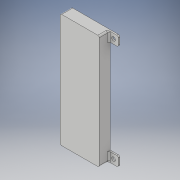
# Autodesk Inventor part: Supporter
Saved by Autodesk Inventor 2018 (Build 220112000, 112)
## iProperties
Created: 2017-12-13
Part Number: Supporter
Material: Generic
Document SubType Name: Modeling
Designer: kcmat
Density: 1 g/cm^3
Appearance: Default
Author: kcmat
Autodesk Inventor part; units mm, degrees
ref_plane "YZ Plane" through (0, 0, 0) normal (1, 0, 0) x (0, 1, 0)
ref_plane "XZ Plane" through (0, 0, 0) normal (0, 1, 0) x (-1, 0, 0)
sketch "Sketch1" plane through (0, 0, 0) normal (0, 0, 1) x (1, 0, 0)
  line L0 (165.7182, 252.0837) -> (146.6642, 252.0837) projected
  line L1 (158.6327, 216.5237) -> (165.7182, 216.5237) projected
  line L2 (139.5562, 216.5237) -> (143.6242, 216.5237) projected
  line L3 (143.6242, 252.0837) -> (139.5562, 252.0837) projected
  line L4 (126.4117, 267.0247) -> (136.1907, 267.0247) projected
  line L5 (136.1907, 190.8247) -> (126.4117, 190.8247) projected
  line L6 (139.5562, 267.0247) -> (139.5562, 190.8247)
  line L7 (139.5562, 190.8247) -> (165.7182, 190.8247)
  line L8 (165.7182, 190.8247) -> (165.7182, 267.0247)
  line L9 (165.7182, 267.0247) -> (139.5562, 267.0247)
  point P0 (0, 0)
  constraints: 8 end point, 3 perpendicular, 1 vertical
ref_plane "Work Plane1" through (146.6642, 216.5237, 7.3936) normal (0, 0, -1) x (0, 1, 0)
extrude "Extrusion1" add sketch "Sketch1" along normal up to surface (7.3936 mm away)
sketch "Sketch2" plane through (0, 0, 0) normal (0, 0, -1) x (-1, 0, 0)
  line L0 (-165.7182, 267.0247) -> (-139.5562, 267.0247) projected
  line L1 (-165.7182, 267.0247) -> (-172.0682, 267.0247)
  line L2 (-172.0682, 267.0247) -> (-172.0682, 260.6747)
  line L3 (-172.0682, 260.6747) -> (-165.7182, 260.6747)
  line L4 (-165.7182, 190.8247) -> (-165.7182, 267.0247) projected
  circle A0 centre (-168.8932, 263.8497) radius 1.25
  line L5 (-165.7182, 228.9247) -> (-182.0836, 228.9247)
  line L6 (-139.5562, 190.8247) -> (-165.7182, 190.8247) projected
  line L7 (-152.6372, 190.8247) -> (-152.6372, 202.3361)
  line L8 (-165.7182, 190.8247) -> (-139.5562, 190.8247)
  line L9 (-165.7182, 190.8247) -> (-172.0682, 190.8247)
  line L10 (-172.0682, 190.8247) -> (-172.0682, 197.1747)
  line L11 (-172.0682, 197.1747) -> (-165.7182, 197.1747)
  line L12 (-165.7182, 267.0247) -> (-165.7182, 190.8247)
  circle A1 centre (-168.8932, 193.9997) radius 1.25
  point P0 (0, 0)
  dimension "d2" = 6.35
  dimension "d3" = 6.35
  dimension "d5" = 2.5
  constraints: 20 end point, 6 symmetric about line, 2 centre point, 2 horizontal, 2 midpoint, 2 point on line, 2 vertical, 1 perpendicular, 1 other
  measures "d2" distance of L0.start L1.end
  measures "d3" distance of L1.end L2.end
  measures "d5" diameter of A0
extrude "Extrusion2" add sketch "Sketch2" against normal blind 1
fillet "Fillet1" radius 1 4 edges at (139.5562, 190.8247, 3.6968) (139.5562, 267.0247, 3.6968) (165.7182, 267.0247, 4.1968) (165.7182, 190.8247, 4.1968)
fillet "Fillet2" radius 1 4 edges at (172.0682, 267.0247, 0.5) (172.0682, 260.6747, 0.5) (172.0682, 197.1747, 0.5) (172.0682, 190.8247, 0.5)
fillet "Fillet3" radius 1 4 edges at (165.4253, 266.7318, 1) (165.7182, 263.3497, 1) (165.4253, 191.1176, 1) (165.7182, 194.4997, 1)
body "Solid1"
